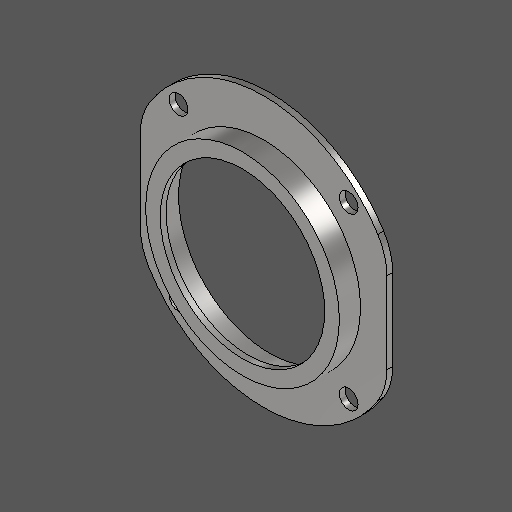
# Autodesk Inventor part: quartz-disk-window-holder
Saved by Autodesk Inventor 2025 (Build 290162000, 162)
## iProperties
Created: 2024-05-22
Part Number: quartz-disk-window-holder
Material: Stainless Steel
Document SubType Name: Modeling
Designer: kuzmin
Density: 8 g/cm^3
Appearance: Semi-Polished
Author: kuzmin
Autodesk Inventor part; units mm, degrees
ref_plane "YZ Plane" through (0, 0, 0) normal (1, 0, 0) x (0, 1, 0)
ref_plane "XZ Plane" through (0, 0, 0) normal (0, 1, 0) x (-1, 0, 0)
ref_plane "XY Plane" through (0, 0, 0) normal (0, 0, 1) x (1, 0, 0)
sketch "Sketch1" plane through (0, 0, 0) normal (0, 1, 0) x (-1, 0, 0)
  line L0 (0, 0) -> (0, 4.6)
  line L1 (0, 4.6) -> (14, 4.6) construction
  line L2 (14, 4.6) -> (16.5, 4.6)
  line L3 (16.5, 4.6) -> (16.5, 1)
  line L4 (16.5, 1) -> (23, 1)
  line L5 (23, 1) -> (23, 0)
  line L6 (23, 0) -> (15.5, 0)
  line L7 (15.5, 0) -> (0, 0) construction
  line L8 (14, 4.6) -> (14, 3.6)
  line L9 (14, 3.6) -> (15.5, 3.6)
  line L10 (15.5, 3.6) -> (15.5, 0)
  dimension "d0" = 46
  dimension "d2" = 31
  dimension "d3" = 28
  dimension "d4" = 3.6
  dimension "d5" = 1
  dimension "d6" = 1
  dimension "d7" = 1
  constraints: 23 end point, 8 perpendicular, 2 vertical, 1 point on line
  measures "d0" diameter of L5 L0
  measures "d2" diameter of L10 L0
  measures "d3" diameter of L8 L0
  measures "d4" distance of L9.end L6.end
  measures "d5" distance of L1.end L8.end
  measures "d6" distance between parallel lines of L3 L10
  measures "d7" distance of L4.end L5.end
revolve "Revolution1" add sketch "Sketch1" angle 360 about axis through (0, 0, 0) along (0, 0, 1)
sketch "Sketch2" plane through (0, 0, 1) normal (0, 0, 1) x (1, 0, 0)
  circle A0 centre (0, 0) radius 20.5 construction
  line L0 (-14.4957, 14.4957) -> (0, 0) construction
  line L1 (0, 0) -> (-12.5096, 0) construction
  dimension "d9" = 41
  dimension "d20" = 45
  constraints: 4 end point, 1 coincident, 1 horizontal, 3 other
  measures "d20" angle of L1 L0
hole "Hole1" at (-14.4957, 14.4957, 1) direction (0, 0, -1) diameter 3.2 end through all
pattern_circular "Circular Pattern1" count 4 over 360 about axis through (0, 0, 0.5) along (0, 0, 1) of "Hole1"
sketch "Sketch3" plane through (0, 0, 0) normal (0, 0, 1) x (1, 0, 0)
  line L0 (-28.4447, -15.8605) -> (-21, -15.8605)
  line L1 (-21, -15.8605) -> (-21, 15.8605)
  line L2 (-21, 15.8605) -> (-28.4447, 15.8605)
  line L3 (-28.4447, 15.8605) -> (-28.4447, -15.8605)
  point P0 (0, 0)
  point P1 (-28.4447, 0)
  dimension "d21" = 21
  constraints: 8 end point, 2 parallel, 1 horizontal, 1 horizontal alignment, 1 midpoint, 1 perpendicular
  measures "d21" distance from line of point (0, 0) L1
extrude "Extrusion1" cut sketch "Sketch3" along normal through all
fillet "Fillet1" radius 10 2 edges at (-21, -9.3808, 0.5) (-21, 9.3808, 0.5)
mirror "Mirror1" about plane through (0, 0, 0) normal (1, 0, 0) of "Extrusion1", "Fillet1"
equation "\"d5\" = wall_thickness"
equation "\"d6\" = wall_thickness"
equation "\"d7\" = wall_thickness"
equation "\"wall_thickness\" = 1"
body "Solid1"
